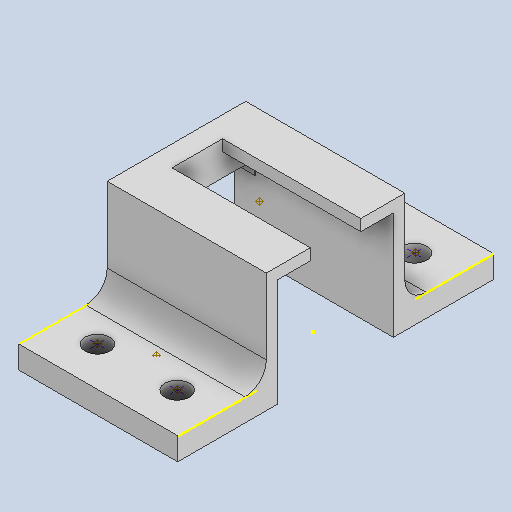
# Autodesk Inventor part: peltierclip_ledgereod2
Saved by Autodesk Inventor 2024.2 (Build 282272000, 272)
## iProperties
Created: 2023-03-14
Part Number: peltierclip_ledgereod2
Material: Generic
Document SubType Name: Modeling
Designer: warke
Density: 1 g/cm^3
Appearance: Default
Author: warke
Autodesk Inventor part; units mm, degrees
ref_plane "YZ Plane" through (0, 0, 0) normal (1, 0, 0) x (0, 1, 0)
ref_plane "XZ Plane" through (0, 0, 0) normal (0, 1, 0) x (-1, 0, 0)
ref_plane "XY Plane" through (0, 0, 0) normal (0, 0, 1) x (1, 0, 0)
sketch "Sketch1" plane through (0, 0, 0) normal (1, 0, 0) x (0, 1, 0)
  line L0 (2.5, 8) -> (-2.5, -8) construction
  line L1 (-2.5, 8) -> (2.5, -8) construction
  line L2 (2.5, 8) -> (2.5, 3.55)
  line L3 (2.5, -8) -> (2.5, -3.55)
  line L4 (-2.5, 0) -> (0.675, 0)
  line L5 (2.5, 8) -> (8.85, 8)
  line L6 (8.85, 8) -> (8.85, -8)
  line L7 (8.85, -8) -> (2.5, -8)
  arc A0 (2.5, -3.55) -> (2.5, 3.55) centre (0.675, 0) ccw
  line L8 (2.5, -8) -> (2.5, -3.55)
  line L9 (2.5, 3.55) -> (2.5, 8)
  point P0 (0, 0)
  dimension "d0" = 5
  dimension "d1" = 16
  dimension "d2" = 4.45
  dimension "d4" = 3.175
  dimension "d7" = 6.35
  constraints: 20 end point, 2 horizontal, 2 midpoint, 2 perpendicular, 2 point on circle, 1 centre point
  measures "d0" distance of L1.end L0.end
  measures "d1" distance of L0.end L1.start
  measures "d2" distance of L2.end L0.start
  measures "d4" distance of L4.start L4.end
  measures "d7" distance of L0.start L5.end
extrude "Extrusion1" add sketch "Sketch1" along normal blind 3.175
sketch "Sketch2" plane through (0, 0, 0) normal (-1, 0, 0) x (0, 0, 1)
  line L0 (-8, 8.85) -> (8, 8.85) projected
  line L1 (8, 2.5) -> (3.55, 2.5) projected
  line L2 (-8, 8.85) -> (8, 8.85)
  line L3 (8, 8.85) -> (8, 2.5)
  line L4 (8, 2.5) -> (-8, 2.5)
  line L5 (-8, 2.5) -> (-8, 8.85)
  point P0 (0, 0)
  constraints: 8 end point, 2 parallel, 1 horizontal, 1 perpendicular
extrude "Extrusion2" add sketch "Sketch2" along normal blind 16
sketch "Sketch3" plane through (-16, 0, 0) normal (-1, 0, 0) x (0, 0, 1)
  line L0 (-8, 2.5) -> (-8, 8.85) projected
  line L1 (8, 2.5) -> (3.55, 2.5) projected
  line L2 (-8, 8.85) -> (8, 8.85)
  line L3 (8, 8.85) -> (8, 2.5)
  line L4 (8, 2.5) -> (-8, 2.5)
  line L5 (-8, 2.5) -> (-8, 8.85)
  point P0 (0, 0)
  constraints: 8 end point, 2 parallel, 1 horizontal, 1 perpendicular
extrude "Extrusion3" add sketch "Sketch3" along normal blind 3.175
sketch "Sketch4" plane through (3.175, 2.5, 3.55) normal (0, -1, 0) x (1, 0, 0)
  line L0 (-22.35, -11.55) -> (-22.35, 4.45) projected
  line L1 (-3.175, -7.1) -> (0, -7.1) projected
  line L2 (-19.175, 0) -> (-3.175, 0)
  line L3 (-3.175, 0) -> (-3.175, -7.1)
  line L4 (-3.175, -7.1) -> (-19.175, -7.1)
  line L5 (-19.175, -7.1) -> (-19.175, 0)
  line L6 (-19.175, 0) -> (-3.175, -7.1) construction
  line L7 (-3.175, 0) -> (-19.175, -7.1) construction
  point P0 (-3.175, -3.55)
  constraints: 12 end point, 2 parallel, 1 horizontal, 1 perpendicular
extrude "Extrusion4" cut sketch "Sketch4" against normal through all
sketch "Sketch5" plane through (-16, 2.5, 3.55) normal (1, 0, 0) x (0, 0, -1)
  line L0 (0, 6.35) -> (7.1, 6.35) projected
  line L1 (0, 0) -> (7.1, 0)
  line L2 (7.1, 0) -> (7.1, 6.35)
  line L3 (7.1, 6.35) -> (0, 6.35)
  line L4 (0, 6.35) -> (0, 0)
  point P0 (3.55, -2.5)
  constraints: 8 end point, 2 parallel, 1 horizontal, 1 perpendicular
extrude "Extrusion5" cut sketch "Sketch5" against normal blind 0.25
sketch "Sketch6" plane through (0, 0.675, 0) normal (-1, 0, 0) x (0, 0, 1)
  line L0 (-3.55, 1.825) -> (-3.55, 8.175) projected
  line L1 (3.55, 1.825) -> (3.55, 8.175) projected
  line L2 (-3.55, 1.825) -> (3.55, 1.825)
  line L3 (3.55, 1.825) -> (3.55, 8.175)
  line L4 (3.55, 8.175) -> (-3.55, 8.175)
  line L5 (-3.55, 8.175) -> (-3.55, 1.825)
  point P0 (0, -0.675)
  constraints: 8 end point, 2 parallel, 1 horizontal, 1 perpendicular
extrude "Extrusion6" cut sketch "Sketch6" against normal blind 0.25
sketch "Sketch7" plane through (3.175, 2.5, 8) normal (0, 0, 1) x (1, 0, 0)
  line L0 (-22.35, 6.35) -> (0, 6.35)
  line L1 (0, 6.35) -> (0, 0)
  line L2 (0, 0) -> (-22.35, 0)
  line L3 (-22.35, 0) -> (-22.35, 6.35)
  point P0 (-3.175, -2.5)
  constraints: 8 end point, 2 parallel, 1 horizontal, 1 perpendicular
extrude "Extrusion7" add sketch "Sketch7" along normal blind 3.175
sketch "Sketch8" plane through (3.175, 2.5, -8) normal (0, 0, -1) x (-1, 0, 0)
  line L0 (0, 6.35) -> (22.35, 6.35) projected
  line L1 (22.35, 6.35) -> (22.35, 0) projected
  line L2 (0, 6.35) -> (22.35, 6.35)
  line L3 (22.35, 6.35) -> (22.35, 0)
  line L4 (22.35, 0) -> (0, 0)
  line L5 (0, 0) -> (0, 6.35)
  point P0 (3.175, -2.5)
  constraints: 8 end point, 2 parallel, 1 horizontal, 1 perpendicular
extrude "Extrusion8" add sketch "Sketch8" along normal blind 3.175
sketch "Sketch9" plane through (-16.25, 2.5, -3.55) normal (0, -1, 0) x (1, 0, 0)
  line L0 (19.425, -7.625) -> (-2.925, -7.625) projected
  line L1 (-2.925, 14.725) -> (-2.925, -7.625) projected
  line L2 (19.425, -7.625) -> (-2.925, -7.625)
  line L3 (-2.925, -7.625) -> (-2.925, -4.45)
  line L4 (-2.925, -4.45) -> (19.425, -4.45)
  line L5 (19.425, -4.45) -> (19.425, -7.625)
  line L6 (19.425, 7.1) -> (19.425, 14.725) projected
  line L7 (-2.925, 14.725) -> (19.425, 14.725)
  line L8 (19.425, 14.725) -> (19.425, 11.55)
  line L9 (19.425, 11.55) -> (-2.925, 11.55)
  line L10 (-2.925, 11.55) -> (-2.925, 14.725)
  point P0 (16.25, 3.55)
  dimension "d26" = 3.175
  dimension "d27" = 3.175
  constraints: 16 end point, 4 parallel, 2 horizontal, 2 perpendicular, 2 point on line
  measures "d26" distance of L2.end L3.end
  measures "d27" distance of L7.end L8.end
extrude "Extrusion9" add sketch "Sketch9" along normal blind 15.142
sketch "Sketch10" plane through (3.175, 2.5, 11.175) normal (0, 0, 1) x (1, 0, 0)
  line L0 (0, -15.142) -> (-22.35, -15.142) projected
  line L1 (0, 0) -> (0, -15.142) projected
  line L2 (-22.35, -15.142) -> (0, -15.142)
  line L3 (0, -15.142) -> (0, -11.967)
  line L4 (0, -11.967) -> (-22.35, -11.967)
  line L5 (-22.35, -11.967) -> (-22.35, -15.142)
  point P0 (-3.175, -2.5)
  dimension "d30" = 3.175
  constraints: 8 end point, 2 parallel, 1 horizontal, 1 perpendicular, 1 point on line
  measures "d30" distance of L3.end L2.end
extrude "Extrusion10" add sketch "Sketch10" along normal blind 5.715
sketch "Sketch11" plane through (3.175, 2.5, -11.175) normal (0, 0, -1) x (-1, 0, 0)
  line L0 (22.35, -15.142) -> (0, -15.142) projected
  line L1 (22.35, 0) -> (22.35, -15.142) projected
  line L2 (0, -15.142) -> (22.35, -15.142)
  line L3 (22.35, -15.142) -> (22.35, -11.967)
  line L4 (22.35, -11.967) -> (0, -11.967)
  line L5 (0, -11.967) -> (0, -15.142)
  point P0 (3.175, -2.5)
  dimension "d33" = 3.175
  constraints: 8 end point, 2 parallel, 1 horizontal, 1 perpendicular, 1 point on line
  measures "d33" distance of L3.end L2.end
extrude "Extrusion11" add sketch "Sketch11" along normal blind 5.715
chamfer "Chamfer1" [suppressed]
sketch "Sketch14" plane through (3.175, 2.5, 16.89) normal (0, 0, 1) x (1, 0, 0)
  line L0 (0, -11.967) -> (-22.35, -11.967) projected
  line L1 (0, 0) -> (0, -15.142) projected
  line L2 (-22.35, -11.967) -> (0, -11.967)
  line L3 (0, -11.967) -> (0, -15.142)
  line L4 (0, -15.142) -> (-22.35, -15.142)
  line L5 (-22.35, -15.142) -> (-22.35, -11.967)
  point P0 (-3.175, -2.5)
  constraints: 8 end point, 2 parallel, 1 horizontal, 1 perpendicular
extrude "Extrusion12" add sketch "Sketch14" along normal blind 5.285
sketch "Sketch15" plane through (3.175, 2.5, -16.89) normal (0, 0, -1) x (-1, 0, 0)
  line L0 (0, -11.967) -> (0, -15.142) projected
  line L1 (0, -15.142) -> (22.35, -15.142) projected
  line L2 (0, -11.967) -> (22.35, -11.967)
  line L3 (22.35, -11.967) -> (22.35, -15.142)
  line L4 (22.35, -15.142) -> (0, -15.142)
  line L5 (0, -15.142) -> (0, -11.967)
  point P0 (3.175, -2.5)
  constraints: 8 end point, 2 parallel, 1 horizontal, 1 perpendicular
extrude "Extrusion13" add sketch "Sketch15" along normal blind 5.285
sketch "Sketch16" plane through (-19.175, -9.467, -11.175) normal (0, 1, 0) x (1, 0, 0)
  point P0 (19.175, -11.175)
chamfer "Chamfer2" distance 3 angle 45 2 edges at (-8, 8.85, 11.175) (-8, 8.85, -11.175)
sketch "Sketch20" plane through (-19.175, 2.5, -8) normal (0, 0, 1) x (1, 0, 0)
  line L0 (0, -15.142) -> (22.35, -15.142)
  line L1 (22.35, -15.142) -> (22.35, 0)
  line L2 (22.35, 0) -> (0, 0)
  line L3 (0, 0) -> (0, -15.142)
  point P0 (19.175, -2.5)
  constraints: 8 end point, 2 parallel, 1 horizontal, 1 perpendicular
extrude "Extrusion17" cut sketch "Sketch20" against normal blind 0.125
sketch "Sketch21" plane through (3.175, 2.5, 8) normal (0, 0, -1) x (-1, 0, 0)
  line L0 (22.35, 0) -> (22.35, -15.142) projected
  line L1 (0, 0) -> (0, -15.142) projected
  line L2 (22.35, -15.142) -> (0, -15.142)
  line L3 (0, -15.142) -> (0, 0)
  line L4 (0, 0) -> (22.35, 0)
  line L5 (22.35, 0) -> (22.35, -15.142)
  point P0 (3.175, -2.5)
  point P1 (0, -15.142)
  constraints: 8 end point, 2 parallel, 1 horizontal, 1 perpendicular
extrude "Extrusion18" cut sketch "Sketch21" against normal blind 0.125
sketch "Sketch22" plane through (-19.175, 8.85, -8.175) normal (0, 1, 0) x (1, 0, 0)
  line L0 (19.425, -11.725) -> (22.35, -11.725) projected
  line L1 (19.425, -4.625) -> (22.35, -4.625) projected
  line L2 (19.425, -11.725) -> (22.35, -11.725)
  line L3 (22.35, -11.725) -> (22.35, -4.625)
  line L4 (22.35, -4.625) -> (19.425, -4.625)
  line L5 (19.425, -4.625) -> (19.425, -11.725)
  point P0 (19.175, -8.175)
  constraints: 8 end point, 2 parallel, 1 horizontal, 1 perpendicular
extrude "Extrusion19" cut sketch "Sketch22" against normal through all
sketch "Sketch23" plane through (-19.175, -9.467, 11.175) normal (0, 1, 0) x (1, 0, 0)
  line L0 (0, 0) -> (0, -11) projected
  line L1 (22.35, 0) -> (22.35, -11) projected
  point P0 (19.175, 11.175)
  point P1 (5.575, -5.5)
  point P2 (16.775, -5.5)
sketch "Sketch24" plane through (-19.175, -9.467, -11.175) normal (0, 1, 0) x (1, 0, 0)
  line L0 (22.35, 0) -> (22.35, 11) projected
  line L1 (0, 0) -> (0, 11) projected
  point P0 (19.175, -11.175)
  point P1 (16.775, 5.5)
  point P2 (5.575, 5.5)
hole "Hole1" at (-13.6, -9.467, -16.675) direction (0, -1, 0) diameter 3.454 end through all clearance for "Flat Head Machine Screw (82)" size "#4" standard "Ansi Unified Screw Threads"
hole "Hole2" at (-2.4, -9.467, -16.675) direction (0, -1, 0) diameter 3.454 end through all clearance for "Flat Head Machine Screw (82)" size "#4" standard "Ansi Unified Screw Threads"
hole "Hole3" at (-2.4, -9.467, 16.675) direction (0, -1, 0) diameter 3.454 end through all clearance for "Flat Head Machine Screw (82)" size "#4" standard "Ansi Unified Screw Threads"
hole "Hole4" at (-13.6, -9.467, 16.675) direction (0, -1, 0) diameter 3.454 end through all clearance for "Flat Head Machine Screw (82)" size "#4" standard "Ansi Unified Screw Threads"
sketch "Sketch25" plane through (3.175, 0, 0) normal (1, 0, 0) x (0, 0, -1)
  line L0 (3.55, 5.0908) -> (8.175, 5.0908)
  line L1 (8.175, 8.85) -> (-8.175, 8.85) projected
  line L2 (8.175, 5.0908) -> (8.175, 8.85)
  line L3 (8.175, 8.85) -> (3.55, 8.85)
  line L4 (3.55, 8.85) -> (8.175, 8.85)
  line L5 (8.175, 8.85) -> (8.175, 5.0908)
  line L6 (8.175, 5.0908) -> (3.55, 5.0908)
  line L7 (3.55, 5.0908) -> (3.55, 8.85)
  point P0 (0, 0)
  point P1 (3.55, 2.5)
  dimension "d102" = 2.5908
  constraints: 14 end point, 2 horizontal, 2 parallel, 2 perpendicular, 1 collinear
  measures "d102" distance of point (3.55, 2.5) L0.start
extrude "Extrusion20" [suppressed]
chamfer "Chamfer3" [suppressed]
sketch "Sketch26" plane through (3.175, 0, 0) normal (1, 0, 0) x (0, 0, -1)
  line L0 (3.55, 2.5) -> (-3.55, 2.5) projected
  line L1 (-3.55, 2.5) -> (-3.55, 5.675)
  line L2 (-3.55, 2.5) -> (-3.55, 8.85) projected
  line L3 (-3.55, 5.675) -> (-11.175, 5.675)
  line L4 (-11.175, 5.85) -> (-11.175, -9.467) projected
  line L5 (-11.175, 5.85) -> (-8.175, 8.85)
  line L6 (-8.175, 8.85) -> (-3.55, 8.85)
  line L7 (3.55, 8.85) -> (3.55, 2.5) projected
  line L8 (3.55, 2.5) -> (3.55, 5.675)
  line L9 (3.55, 5.675) -> (11.175, 5.675)
  line L10 (11.175, 5.85) -> (11.175, -9.467) projected
  line L11 (11.175, 5.85) -> (8.175, 8.85)
  line L12 (11.175, 5.85) -> (8.175, 8.85) projected
  line L13 (8.175, 8.85) -> (3.55, 8.85)
  line L14 (3.55, 8.85) -> (3.55, 5.675)
  point P0 (0, 0)
  dimension "d109" = 3.175
  dimension "d110" = 3.175
  constraints: 18 end point, 3 point on line, 2 midpoint, 2 parallel, 2 perpendicular, 1 collinear, 1 horizontal
  measures "d109" distance of L0.end L1.end
  measures "d110" distance of L0.start L8.end
extrude "Extrusion21" cut sketch "Sketch26" against normal through all
sketch "Sketch27" plane through (-19.175, 8.85, -3.55) normal (0, 1, 0) x (1, 0, 0)
  line L0 (2.925, 0) -> (2.925, -7.1) projected
  line L1 (0, 0) -> (2.925, 0)
  line L2 (2.925, 0) -> (2.925, -7.1)
  line L3 (2.925, -7.1) -> (0, -7.1)
  line L4 (0, -7.1) -> (0, 0)
  point P0 (19.175, -3.55)
  constraints: 8 end point, 2 parallel, 1 horizontal, 1 perpendicular
extrude "Extrusion22" cut sketch "Sketch27" against normal blind 3.175
sketch "Sketch28" plane through (-16.25, 2.5, -3.55) normal (0, -1, 0) x (1, 0, 0)
  line L0 (-2.925, 11.675) -> (-2.925, -4.575) projected
  line L1 (-2.925, -4.575) -> (19.425, -4.575) projected
  line L2 (-2.925, 11.675) -> (0, 11.675)
  line L3 (0, 11.675) -> (0, -4.575)
  line L4 (0, -4.575) -> (-2.925, -4.575)
  line L5 (-2.925, -4.575) -> (-2.925, 11.675)
  point P0 (16.25, 3.55)
  dimension "d115" = 2.925
  constraints: 8 end point, 2 parallel, 1 horizontal, 1 perpendicular, 1 point on line
  measures "d115" distance of L3.end L4.end
extrude "Extrusion23" add sketch "Sketch28" along normal blind 3.175
chamfer "Chamfer4" [suppressed]
sketch "Sketch29" plane through (-16.25, -12.642, -3.55) normal (0, -1, 0) x (1, 0, 0)
  line L0 (-2.925, 11.675) -> (19.425, 11.675) projected
  line L1 (19.425, -4.575) -> (-2.925, -4.575) projected
  line L2 (19.425, 11.675) -> (-2.925, 11.675)
  line L3 (-2.925, 11.675) -> (-2.925, -4.575)
  line L4 (-2.925, -4.575) -> (19.425, -4.575)
  line L5 (19.425, -4.575) -> (19.425, 11.675)
  point P0 (16.25, 3.55)
  constraints: 8 end point, 2 parallel, 1 horizontal, 1 perpendicular
extrude "Extrusion24" [suppressed]
sketch "Sketch30" plane through (-16.25, -12.642, -3.55) normal (0, -1, 0) x (1, 0, 0)
  line L0 (-2.925, 11.675) -> (19.425, 11.675) projected
  line L1 (-2.925, -4.575) -> (-2.925, -18.625) projected
  line L2 (19.425, 11.675) -> (-2.925, 11.675)
  line L3 (-2.925, 11.675) -> (-2.925, -4.575)
  line L4 (-2.925, -4.575) -> (19.425, -4.575)
  line L5 (19.425, -4.575) -> (19.425, 11.675)
  point P0 (16.25, 3.55)
  constraints: 8 end point, 2 parallel, 1 horizontal, 1 perpendicular
extrude "Extrusion25" [suppressed]
sketch "Sketch31" plane through (3.175, 5.675, 11.175) normal (0, 1, 0) x (1, 0, 0)
  line L0 (-19.425, 14.725) -> (-19.425, 7.625) projected
  line L1 (0, 14.725) -> (-19.425, 14.725)
  line L2 (-19.425, 14.725) -> (-19.425, 7.625)
  line L3 (-19.425, 7.625) -> (0, 7.625) projected
  line L4 (-19.425, 7.625) -> (0, 7.625)
  line L5 (0, 7.625) -> (0, 0)
  line L6 (0, 0) -> (-22.35, 0) projected
  line L7 (0, 0) -> (-22.35, 0)
  line L8 (-22.35, 0) -> (-22.35, 22.35) projected
  line L9 (-22.35, 0) -> (-22.35, 22.35)
  line L10 (-22.35, 22.35) -> (0, 22.35)
  line L11 (0, 22.35) -> (0, 14.725)
  point P0 (-3.175, 11.175)
  constraints: 16 end point, 4 perpendicular, 3 collinear, 1 horizontal
extrude "Extrusion26" cut sketch "Sketch31" against normal blind 0.5
sketch "Sketch32" plane through (3.175, 5.175, 11.175) normal (0, 1, 0) x (1, 0, 0)
  line L0 (0, 22.35) -> (-22.35, 22.35) projected
  line L1 (-22.35, 0) -> (0, 0) projected
  line L2 (-22.35, 22.35) -> (0, 22.35)
  line L3 (0, 22.35) -> (0, 0)
  line L4 (0, 0) -> (-22.35, 0)
  line L5 (-22.35, 0) -> (-22.35, 22.35)
  point P0 (-3.175, 11.175)
  constraints: 8 end point, 2 parallel, 1 horizontal, 1 perpendicular
extrude "Extrusion27" cut sketch "Sketch32" against normal blind 1.075
sketch "Sketch33" plane through (3.175, 2.5, 11.175) normal (0, 0, 1) x (1, 0, 0)
  line L0 (-22.35, 1.6) -> (0, 1.6) projected
  line L1 (0, -11.967) -> (0, -15.142) projected
  line L2 (-22.35, 1.6) -> (0, 1.6)
  line L3 (0, 1.6) -> (0, -11.967)
  line L4 (0, -11.967) -> (-22.35, -11.967)
  line L5 (-22.35, -11.967) -> (-22.35, 1.6)
  point P0 (-3.175, -2.5)
  constraints: 8 end point, 2 parallel, 1 horizontal, 1 perpendicular
extrude "Extrusion28" cut sketch "Sketch33" against normal blind 1.45
sketch "Sketch34" plane through (3.175, 2.5, -11.175) normal (0, 0, -1) x (-1, 0, 0)
  line L0 (0, -11.967) -> (22.35, -11.967) projected
  line L1 (22.35, 1.6) -> (0, 1.6) projected
  line L2 (22.35, -11.967) -> (0, -11.967)
  line L3 (0, -11.967) -> (0, 1.6)
  line L4 (0, 1.6) -> (22.35, 1.6)
  line L5 (22.35, 1.6) -> (22.35, -11.967)
  point P0 (3.175, -2.5)
  constraints: 8 end point, 2 parallel, 1 horizontal, 1 perpendicular
extrude "Extrusion29" cut sketch "Sketch34" against normal blind 1.45
fillet "Fillet1" radius 3 2 edges at (-8, -9.467, 9.725) (-8, -9.467, -9.725)
fillet "Fillet2" radius 2 2 edges at (-17.7125, -0.675, -8.125) (-17.7125, -0.675, 8.125)
body "Solid1"
